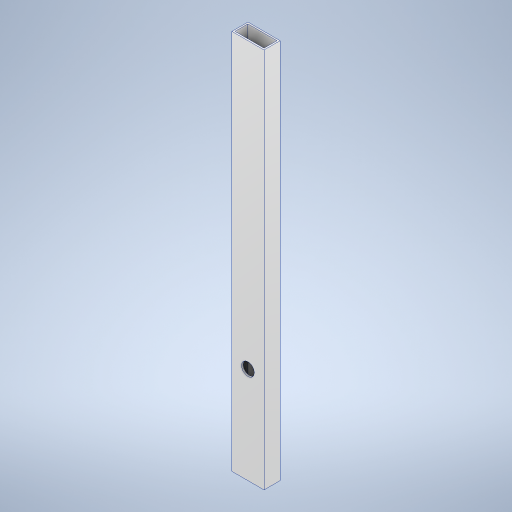
# Autodesk Inventor part: 射出_腕
Saved by Autodesk Inventor 2023 (Build 270158000, 158)
## iProperties
Created: 2022-04-20
Part Number: 射出_腕
Material: アルミニウム 6061
Document SubType Name: Modeling
Designer: yuta
Density: 2.7 g/cm^3
Appearance: アルミニウム - フラット
Author: yuta
Autodesk Inventor part; units mm, degrees
ref_plane "YZ Plane" through (0, 0, 0) normal (1, 0, 0) x (0, 1, 0)
ref_plane "XZ Plane" through (0, 0, 0) normal (0, 1, 0) x (-1, 0, 0)
ref_plane "XY Plane" through (0, 0, 0) normal (0, 0, 1) x (1, 0, 0)
sketch "スケッチ1" plane through (0, 0, 0) normal (0, 1, 0) x (-1, 0, 0)
  line L0 (0, 0) -> (30, 0)
  line L1 (30, 0) -> (30, -15)
  line L2 (30, -15) -> (0, -15)
  line L3 (0, -15) -> (0, 0)
  dimension "d0" = 30
  dimension "d1" = 15
  constraints: 8 end point, 2 parallel, 1 horizontal, 1 perpendicular
  measures "d0" distance of L1.end L2.end
  measures "d1" distance of L0.end L1.end
extrude "押し出し1" add sketch "スケッチ1" along normal blind 300
sketch "スケッチ2" plane through (-30, 0, 0) normal (0, 0, 1) x (1, 0, 0)
  circle A0 centre (15, 45) radius 5
  line L0 (0, 0) -> (30, 0) projected
  line L1 (30, 0) -> (30, 300) projected
  dimension "d4" = 10
  dimension "d5" = 45
  dimension "d6" = 15
  constraints: 1 centre point
  measures "d4" diameter of A0
  measures "d5" distance from line of L0 A0.centre
  measures "d6" distance from line of L1 A0.centre
extrude "押し出し2" cut sketch "スケッチ2" against normal blind 300
sketch "スケッチ3" plane through (0, 0, 0) normal (0, -1, 0) x (1, 0, 0)
  line L0 (-30, 0) -> (0, 0) projected
  line L1 (0, 0) -> (-30, 0)
  line L2 (-30, 0) -> (-30, -15)
  line L3 (-30, -15) -> (0, -15)
  line L4 (0, -15) -> (0, 0)
  dimension "d9" = 30
  dimension "d10" = 15
  constraints: 8 end point, 2 parallel, 1 horizontal, 1 perpendicular
  measures "d9" distance of L3.end L2.end
  measures "d10" distance of L2.end L1.end
extrude "押し出し3" cut sketch "スケッチ3" against normal blind 10
sketch "スケッチ5" plane through (0, 300, 0) normal (0, 1, 0) x (1, 0, 0)
  line L0 (0, 0) -> (0, 15) projected
  line L1 (0, 15) -> (-30, 15) projected
  line L2 (0, 0) -> (-30, 0)
  line L3 (-30, 0) -> (-30, 15)
  line L4 (-30, 15) -> (0, 15)
  line L5 (0, 15) -> (0, 0)
  constraints: 8 end point, 2 parallel, 1 horizontal, 1 perpendicular
extrude "押し出し4" add sketch "スケッチ5" along normal blind 10
sketch "スケッチ6" plane through (0, 10, 0) normal (0, -1, 0) x (1, 0, 0)
  line L0 (0, 0) -> (-30, 0)
  line L1 (-30, 0) -> (-30, -15)
  line L2 (-30, -15) -> (0, -15)
  line L3 (0, -15) -> (0, 0)
  constraints: 8 end point, 2 parallel, 1 horizontal, 1 perpendicular
extrude "押し出し5" add sketch "スケッチ6" along normal blind 60
sketch "スケッチ7" plane through (0, -50, 0) normal (0, -1, 0) x (1, 0, 0)
  line L0 (0, 0) -> (0, -15) projected
  line L1 (0, -15) -> (-30, -15) projected
  line L2 (0, 0) -> (-30, 0)
  line L3 (-30, 0) -> (-30, -15)
  line L4 (-30, -15) -> (0, -15)
  line L5 (0, -15) -> (0, 0)
  constraints: 8 end point, 2 parallel, 1 horizontal, 1 perpendicular
extrude "押し出し6" cut sketch "スケッチ7" against normal blind 5
sketch "スケッチ8" plane through (-30, 310, 0) normal (0, 0, 1) x (1, 0, 0)
  circle A0 centre (15, -265) radius 6
  line L0 (0, -355) -> (30, -355) projected
  line L1 (0, -355) -> (0, 0) projected
  circle A1 centre (15, -265) radius 5
  point P0 (30, -310)
  dimension "d19" = 12
  dimension "d20" = 90
  dimension "d21" = 15
  dimension "d22" = 10
  constraints: 2 centre point, 1 coincident
  measures "d19" diameter of A0
  measures "d20" distance from line of L0 A0.centre
  measures "d21" distance from line of L1 A0.centre
  measures "d22" diameter of A1
extrude "押し出し7" cut sketch "スケッチ8" against normal blind 15
sketch "スケッチ9" plane through (0, 310, 0) normal (0, 1, 0) x (1, 0, 0)
  line L0 (-28.5, 13.5) -> (-1.5, 13.5)
  line L1 (-1.5, 13.5) -> (-1.5, 1.5)
  line L2 (-1.5, 1.5) -> (-28.5, 1.5)
  line L3 (-28.5, 1.5) -> (-28.5, 13.5)
  line L4 (0, 15) -> (-30, 15) projected
  line L5 (-30, 15) -> (-30, 0) projected
  point P0 (0, 0)
  dimension "d25" = 27
  dimension "d26" = 12
  dimension "d27" = 1.5
  dimension "d28" = 1.5
  constraints: 8 end point, 2 parallel, 1 horizontal, 1 perpendicular
  measures "d25" distance of L1.end L2.end
  measures "d26" distance of L0.end L1.end
  measures "d27" distance between parallel lines of L4 L0
  measures "d28" distance between parallel lines of L5 L3
extrude "押し出し8" cut sketch "スケッチ9" against normal blind 500
